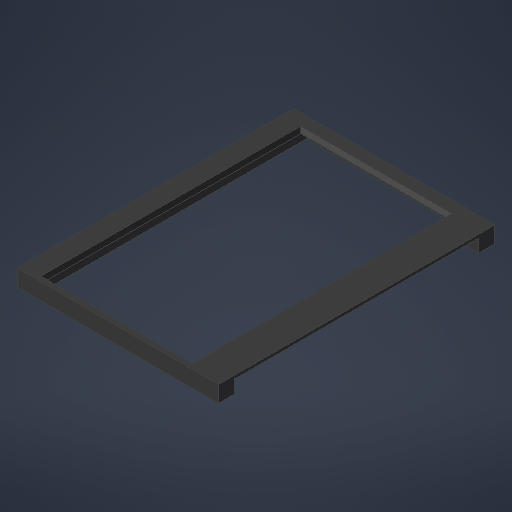
# Autodesk Inventor part: PlantillaPantalla
Saved by Autodesk Inventor 2026.1 (Build 301233020, 233B)
## iProperties
Created: 2025-11-01
Part Number: PlantillaPantalla
Material: Generic
Document SubType Name: Modeling
Designer: Tito Luyo Murata
Density: 1 g/cm^3
Appearance: Default
Author: Tito Luyo Murata
Autodesk Inventor part; units mm, degrees
ref_plane "YZ Plane" through (0, 0, 0) normal (1, 0, 0) x (0, 1, 0)
ref_plane "XZ Plane" through (0, 0, 0) normal (0, 1, 0) x (-1, 0, 0)
ref_plane "XY Plane" through (0, 0, 0) normal (0, 0, 1) x (1, 0, 0)
sketch "Sketch1" plane through (0, 0, 0) normal (0, 1, 0) x (-1, 0, 0)
  line L0 (0, 0) -> (100.5, 0)
  line L1 (100.5, 0) -> (100.5, -165.5)
  line L2 (100.5, -165.5) -> (0, -165.5)
  line L3 (0, -165.5) -> (0, 0)
  line L4 (110.5, 2) -> (-13, 2)
  line L5 (-13, 2) -> (-13, -167.5)
  line L6 (-13, -167.5) -> (110.5, -167.5)
  line L7 (110.5, -167.5) -> (110.5, 2)
  line L8 (110.5, -157.5) -> (102.5, -157.5)
  line L9 (102.5, -157.5) -> (102.5, -8)
  line L10 (102.5, -8) -> (110.5, -8)
  line L11 (110.5, -8) -> (110.5, -157.5)
  line L12 (-13, -157.5) -> (-2, -157.5)
  line L13 (-2, -157.5) -> (-2, -8)
  line L14 (-2, -8) -> (-13, -8)
  line L15 (-13, -8) -> (-13, -157.5)
  point P0 (110.5, -8)
  point P1 (-13, -8)
  dimension "d0" = 100.5
  dimension "d1" = 165.5
  dimension "d2" = 2
  dimension "d3" = 13
  dimension "d4" = 10
  dimension "d5" = 2
  dimension "d33" = 8
  dimension "d34" = 8
  dimension "d35" = 8
  dimension "d36" = 8
  dimension "d37" = 2
  dimension "d38" = 2
  constraints: 32 end point, 8 parallel, 4 horizontal, 4 perpendicular, 2 point on line
  measures "d0" distance of L1.end L2.end
  measures "d1" distance of L0.end L1.end
  measures "d2" distance between parallel lines of L0 L4
  measures "d3" distance between parallel lines of L5 L3
  measures "d4" distance between parallel lines of L7 L1
  measures "d5" distance between parallel lines of L6 L2
  measures "d33" distance between parallel lines of L12 L2
  measures "d34" distance between parallel lines of L8 L2
  measures "d35" distance between parallel lines of L14 L0
  measures "d36" distance between parallel lines of L0 L10
  measures "d37" distance between parallel lines of L13 L3
  measures "d38" distance between parallel lines of L1 L9
extrude "Extrusion1" add sketch "Sketch1" against normal blind 8 contours L7 L10 L9 L8 L6 L5 L12 L13 L14 L4
sketch "Sketch2" plane through (0, 0, 0) normal (0, 1, 0) x (1, 0, 0)
  line L0 (-97, 3) -> (-8, 3)
  line L1 (-8, 3) -> (-8, 158.5)
  line L2 (-8, 158.5) -> (-97, 158.5)
  line L3 (-97, 158.5) -> (-97, 3)
  line L4 (-100.5, 0) -> (-100.5, 165.5) projected
  line L5 (-100.5, 165.5) -> (0, 165.5) projected
  line L6 (0, 165.5) -> (0, 0) projected
  line L7 (0, 0) -> (-100.5, 0) projected
  line L8 (13, -2) -> (-110.5, -2) projected
  line L9 (13, 167.5) -> (13, -2) projected
  line L10 (-110.5, -2) -> (13, -2)
  line L11 (13, -2) -> (13, 167.5)
  line L12 (13, 167.5) -> (-110.5, 167.5)
  line L13 (-110.5, 167.5) -> (-110.5, -2)
  dimension "d8" = 3.5
  dimension "d9" = 7
  dimension "d10" = 8
  dimension "d11" = 3
  constraints: 16 end point, 4 parallel, 2 horizontal, 2 perpendicular
  measures "d8" distance between parallel lines of L4 L3
  measures "d9" distance between parallel lines of L5 L2
  measures "d10" distance between parallel lines of L6 L1
  measures "d11" distance between parallel lines of L7 L0
extrude "Extrusion2" add sketch "Sketch2" along normal blind 2 contours L4 L5 L6 L7 | L8 L13 L12 L9
sketch "Sketch3" plane through (0, -8, 0) normal (0, -1, 0) x (1, 0, 0)
  circle A0 centre (-106, -161.5) radius 1.75
  line L0 (-100.5, -165.5) -> (-100.5, 0) projected
  line L1 (0, -165.5) -> (-100.5, -165.5) projected
  circle A1 centre (-106, -4) radius 1.75
  line L2 (-100.5, 0) -> (0, 0) projected
  circle A2 centre (9.5, -4) radius 1.75
  line L3 (0, 0) -> (0, -165.5) projected
  circle A3 centre (9.5, -161.5) radius 1.75
  dimension "d14" = 3.5
  dimension "d15" = 5.5
  dimension "d16" = 4
  dimension "d17" = 3.5
  dimension "d18" = 4
  dimension "d19" = 5.5
  dimension "d20" = 3.5
  dimension "d21" = 4
  dimension "d22" = 9.5
  dimension "d23" = 3.5
  dimension "d24" = 9.5
  dimension "d25" = 4
  constraints: 4 centre point
  measures "d14" diameter of A0
  measures "d15" distance from line of L0 A0.centre
  measures "d16" distance from line of L1 A0.centre
  measures "d17" diameter of A1
  measures "d18" distance from line of L2 A1.centre
  measures "d19" distance from line of L0 A1.centre
  measures "d20" diameter of A2
  measures "d21" distance from line of L2 A2.centre
  measures "d22" distance from line of L3 A2.centre
  measures "d23" diameter of A3
  measures "d24" distance from line of L3 A3.centre
  measures "d25" distance from line of L1 A3.centre
extrude "Extrusion3" cut sketch "Sketch3" against normal blind 7 contours A0 | A1 | A2 | A3
chamfer "Chamfer1" distance 2 angle 45 4 edges at (-97, 2, -80.75) (-52.5, 2, -3) (-52.5, 2, -158.5) (-8, 2, -80.75)
equation "\"d14\" = hueco_diam"
equation "\"d17\" = hueco_diam"
equation "\"d20\" = hueco_diam"
equation "\"d21\" = hueco_sep_lat"
equation "\"d23\" = hueco_diam"
equation "\"d25\" = hueco_sep_lat"
equation "\"hueco_sep_inf\" = 4.5"
equation "\"hueco_sep_lat\" = 4"
equation "\"tol1\" = 0.5"
equation "\"hueco_diam\" = 3.5"
body "Solid1"
